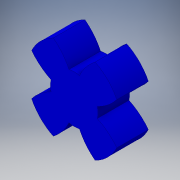
# Autodesk Inventor part: MJT-30-BL Sleeve
Saved by Autodesk Inventor 2019 (Build 230136000, 136)
## iProperties
Created: 2023-09-29
Part Number: MJT-30-BL Sleeve
Material: Generic
Catalog Web Link: www.cadenas.de
Description: MJT Sleeve-
Vendor: NBK
Document SubType Name: Modeling
Designer: psAdmin
Manufacturer: NBK
Mass: 4.70184 g
Surface Area: 21.0625 cm^2
Volume: 4.70184 cm^3
Density: 1 g/cm^3
Appearance: PSOLRGB-0-0-255
Category: PARTsolutions
Company: NBK
Title: MJT-30-BL Sleeve
Author: Cadenas PARTsolutions
PSOL_IDENT_0: {$CADENAS_DATA/23d-libs/nbk/motion_control_parts/couplicon_mini/jaw_type/mjt/mjt_2.prj},176 {VTYP=3D
PSOL_IDENT_1: },{NB=MJT-30-BL Sleeve},{LINA=MJT-30-BL Sleeve},{NN=MJT Sleeve},{DATE=25.09.2023 00:41:45},{GEOMDATE=
PSOL_IDENT_2: 11.08.2014 07:51:00},{VERSION=},{LINEID=30},{WBVAR=},{WBNUMERIC=}  {NB=MJT-30-BL Sleeve},{LINA=MJT-3
PSOL_IDENT_3: 0-BL Sleeve},{KT=DUMMY},{CN=MJT-30-BL},{VERS=1},{A=30},{B=10},{DP=13.22},{DP1=0.00},{COL0R=0.00,0.00
PSOL_IDENT_4: ,1.00,0.00},{E=0.0}
NB: MJT-30-BL Sleeve
NN: MJT Sleeve
NBSYN: $CN. Sleeve
LINA: MJT-30-BL Sleeve
CATALOG: NBK (Nabeya Bi-tech Kaisha
CN: MJT-30-BL
VERS: 1
A: 30
B: 10
DP: 13.22
DP1: 0
COL0R: 0.00,0.00,1.00,0.00
E: 0
SUPPLIER: NBK
ARTICLENO: MJT-30-BL Sleeve
BOMINFO: MJT-30-BL Sleeve
CREATOR: CADENAS GmbH
Autodesk Inventor part; units mm, degrees
sketch "Sketch_1" plane through (0, 0, 0) normal (0, 0, 1) x (1, 0, 0)
  arc A0 (-13.4651, -6.61) -> (-6.61, -13.4651) centre (0, 0) ccw
  arc A1 (-6.61, -13.4651) -> (-1.6525, -7.3157) centre (-17.0197, 0) ccw
  arc A2 (-1.6525, -7.3157) -> (1.6525, -7.3157) centre (0, 0) ccw
  arc A3 (1.6525, -7.3157) -> (6.61, -13.4651) centre (17.0197, 0) ccw
  arc A4 (6.61, -13.4651) -> (13.4651, -6.61) centre (0, 0) ccw
  arc A5 (13.4651, -6.61) -> (7.3157, -1.6525) centre (0, -17.0197) ccw
  arc A6 (7.3157, -1.6525) -> (7.3157, 1.6525) centre (0, 0) ccw
  arc A7 (7.3157, 1.6525) -> (13.4651, 6.61) centre (0, 17.0197) ccw
  arc A8 (13.4651, 6.61) -> (6.61, 13.4651) centre (0, 0) ccw
  arc A9 (6.61, 13.4651) -> (1.6525, 7.3157) centre (17.0197, 0) ccw
  arc A10 (1.6525, 7.3157) -> (-1.6525, 7.3157) centre (0, 0) ccw
  arc A11 (-1.6525, 7.3157) -> (-6.61, 13.4651) centre (-17.0197, 0) ccw
  arc A12 (-6.61, 13.4651) -> (-13.4651, 6.61) centre (0, 0) ccw
  arc A13 (-13.4651, 6.61) -> (-7.3157, 1.6525) centre (0, 17.0197) ccw
  arc A14 (-7.3157, 1.6525) -> (-7.3157, -1.6525) centre (0, 0) ccw
  arc A15 (-7.3157, -1.6525) -> (-13.4651, -6.61) centre (0, -17.0197) ccw
  constraints: 32 point on circle, 16 centre point
extrude "Extrusion1" add sketch "Sketch_1" along normal blind 10
ref_plane "part2a_XY" through (0, 0, 0) normal (0, 0, 1) x (1, 0, 0)
ref_plane "part2a_YZ" through (0, 0, 0) normal (1, 0, 0) x (0, 1, 0)
ref_plane "part2a_ZX" through (0, 0, 0) normal (0, 1, 0) x (0, 0, 1)
body "Solid1"
